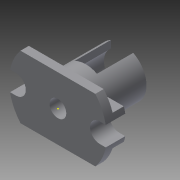
# Autodesk Inventor part: 零件6-23
Saved by Autodesk Inventor 2014 (Build 180170000, 170)
## iProperties
Created: 2018-11-23
Part Number: 零件6-23
Material: 常规
Document SubType Name: Modeling
Designer: Administrator
Density: 1 g/cm^3
Appearance: 默认
Author: Administrator
Autodesk Inventor part; units mm, degrees
ref_plane "YZ Plane" through (0, 0, 0) normal (1, 0, 0) x (0, 1, 0)
ref_plane "XZ Plane" through (0, 0, 0) normal (0, 1, 0) x (-1, 0, 0)
ref_plane "XY Plane" through (0, 0, 0) normal (0, 0, 1) x (1, 0, 0)
sketch "草图1" plane through (0, 0, 0) normal (0, 1, 0) x (-1, 0, 0)
  line L0 (55.7629, 0) -> (-64.7988, 0)
  line L1 (26.8095, -22.5) -> (-26.8095, -22.5)
  line L2 (26.8095, 22.5) -> (-29.1705, 22.5)
  line L3 (0, -45.1984) -> (0, 63.6584)
  arc A0 (30, 7) -> (30, -7) centre (30, 0) ccw
  arc A1 (-30, -7) -> (-30, 7) centre (-30, 0) ccw
  line L4 (30, -7) -> (34.2929, -7)
  line L5 (30, 7) -> (34.2929, 7)
  line L6 (-30, -7) -> (-34.2929, -7)
  line L7 (-30, 7) -> (-34.2929, 7)
  arc A2 (26.8095, -22.5) -> (34.2929, -7) centre (0, 0) ccw
  arc A3 (34.2929, 7) -> (26.8095, 22.5) centre (0, 0) ccw
  arc A4 (-26.8095, 22.5) -> (-34.2929, 7) centre (0, 0) ccw
  arc A5 (-34.2929, -7) -> (-26.8095, -22.5) centre (0, 0) ccw
  dimension "d1" = 45
  dimension "d2" = 14
  dimension "d3" = 60
  constraints: 16 end point, 12 point on circle, 6 centre point, 5 parallel, 5 point on line, 4 tangent, 2 perpendicular, 1 coincident, 1 horizontal, 2 other
  measures "d1" diameter of L1 L0
  measures "d2" diameter of A0
  measures "d3" distance of A1.centre A0.centre
extrude "拉伸1" add sketch "草图1" along normal blind 6
sketch "草图2" plane through (0, 6, 0) normal (0, 1, 0) x (1, 0, 0)
  arc A0 (34.2929, 7) -> (26.8095, 22.5) centre (0, 0) ccw projected
  circle A1 centre (0, 0) radius 17.5
  dimension "d6" = 35
  constraints: 1 centre point, 1 coincident
  measures "d6" diameter of A1
extrude "拉伸2" add sketch "草图2" along normal blind 40
sketch "草图3" plane through (0, 0, 0) normal (0, -1, 0) x (1, 0, 0)
  arc A0 (-34.2929, -7) -> (-26.8095, -22.5) centre (0, 0) ccw projected
  circle A1 centre (0, 0) radius 6
  dimension "d9" = 12
  constraints: 1 centre point, 1 coincident
  measures "d9" diameter of A1
extrude "拉伸3" cut sketch "草图3" against normal blind 60
sketch "草图4" plane through (0, 6, 0) normal (0, 1, 0) x (1, 0, 0)
  circle A0 centre (0, 0) radius 17.5 projected
  arc A1 (-26.8095, 22.5) -> (-34.2929, 7) centre (0, 0) ccw projected
  line L0 (-34.2929, 7) -> (-30, 7) projected
  arc A2 (-30, -7) -> (-30, 7) centre (-30, 0) ccw projected
  line L1 (-30, -7) -> (-34.2929, -7) projected
  arc A3 (-34.2929, -7) -> (-26.8095, -22.5) centre (0, 0) ccw projected
  arc A4 (26.8095, -22.5) -> (34.2929, -7) centre (0, 0) ccw projected
  line L2 (34.2929, -7) -> (30, -7) projected
  arc A5 (30, 7) -> (30, -7) centre (30, 0) ccw projected
  line L3 (30, 7) -> (34.2929, 7) projected
  arc A6 (34.2929, 7) -> (26.8095, 22.5) centre (0, 0) ccw projected
  line L4 (-33.2265, 11) -> (-13.6107, 11)
  line L5 (13.6107, 11) -> (33.2265, 11)
  line L6 (-33.2265, -11) -> (-13.6107, -11)
  line L7 (13.6107, -11) -> (33.2265, -11)
  line L8 (-37.479, 0) -> (55.827, 0)
  line L9 (0, 23.5503) -> (0, -22.0958)
  dimension "d12" = 22
  constraints: 12 end point, 8 point on circle, 3 parallel, 1 collinear, 1 perpendicular, 2 other
  measures "d12" diameter of L4 L8
extrude "拉伸4" add sketch "草图4" along normal blind 8 contours L8 A5 L2 A4 L7 A0 | A0 L5 A6 L3 A5 L8 | L8 A2 L0 A1 L4 A0 | A0 L6 A3 L1 A2 L8
sketch "草图5" plane through (0, 46, 0) normal (0, 1, 0) x (1, 0, 0)
  circle A0 centre (0, 0) radius 6 projected
  circle A1 centre (0, 0) radius 17.5 projected
  circle A2 centre (0, 0) radius 13
  dimension "d15" = 26
  constraints: 1 centre point, 1 coincident
  measures "d15" diameter of A2
extrude "拉伸5" cut sketch "草图5" against normal blind 26 contours A2
sketch "草图6" plane through (0, 0, 0) normal (0, 0, 1) x (1, 0, 0)
  point P0 (0, 0)
sketch "草图7" plane through (0, 0, 0) normal (0, 0, 1) x (1, 0, 0)
  line L0 (0, 0) -> (0, 58.8844)
  line L1 (-23, 14) -> (-17.5, 14) projected
  line L2 (-17.5, 14) -> (-17.5, 46) projected
  line L3 (-17.5, 46) -> (-13, 46) projected
  line L4 (-13, 46) -> (-13, 20) projected
  line L5 (-13, 20) -> (-6, 20) projected
  line L6 (-6, 20) -> (-6, 0) projected
  line L7 (-6, 0) -> (-23, 0) projected
  line L8 (-23, 0) -> (-23, 14) projected
  line L9 (17.5, 14) -> (23, 14) projected
  line L10 (23, 14) -> (23, 0) projected
  line L11 (23, 0) -> (6, 0) projected
  line L12 (6, 0) -> (6, 20) projected
  line L13 (6, 20) -> (13, 20) projected
  line L14 (13, 20) -> (13, 46) projected
  line L15 (13, 46) -> (17.5, 46) projected
  line L16 (17.5, 46) -> (17.5, 14) projected
  circle A0 centre (0, 34) radius 8
  line L17 (-13, 46) -> (13, 46) projected
  dimension "d18" = 16
  dimension "d19" = 12
  constraints: 2 end point, 1 centre point, 1 point on line, 1 vertical
  measures "d18" diameter of A0
  measures "d19" distance from line of L17 A0.centre
extrude "拉伸6" cut sketch "草图7" against normal blind 26 contours A0 L0 | L0 A0
sketch "草图8" plane through (0, 0, 0) normal (0, 0, 1) x (1, 0, 0)
  line L0 (-23, 14) -> (-17.5, 14) projected
  line L1 (-17.5, 14) -> (-17.5, 46) projected
  line L2 (-17.5, 46) -> (-13, 46) projected
  line L3 (-13, 46) -> (-13, 20) projected
  line L4 (-13, 20) -> (-6, 20) projected
  line L5 (-6, 20) -> (-6, 0) projected
  line L6 (-6, 0) -> (-23, 0) projected
  line L7 (-23, 0) -> (-23, 14) projected
  line L8 (17.5, 14) -> (23, 14) projected
  line L9 (23, 14) -> (23, 0) projected
  line L10 (23, 0) -> (6, 0) projected
  line L11 (6, 0) -> (6, 20) projected
  line L12 (6, 20) -> (13, 20) projected
  line L13 (13, 20) -> (13, 46) projected
  line L14 (13, 46) -> (17.5, 46) projected
  line L15 (17.5, 46) -> (17.5, 14) projected
  line L16 (-23, 14) -> (-17.5, 14) projected
  line L17 (-17.5, 14) -> (-17.5, 46) projected
  line L18 (-17.5, 46) -> (-13, 46) projected
  line L19 (-13, 46) -> (-13, 20) projected
  line L20 (-13, 20) -> (-6, 20) projected
  line L21 (-6, 20) -> (-6, 0) projected
  line L22 (-6, 0) -> (-23, 0) projected
  line L23 (-23, 0) -> (-23, 14) projected
  line L24 (17.5, 14) -> (23, 14) projected
  line L25 (23, 14) -> (23, 0) projected
  line L26 (23, 0) -> (6, 0) projected
  line L27 (6, 0) -> (6, 20) projected
  line L28 (6, 20) -> (13, 20) projected
  line L29 (13, 20) -> (13, 46) projected
  line L30 (13, 46) -> (17.5, 46) projected
  line L31 (17.5, 46) -> (17.5, 14) projected
  line L32 (-23, 14) -> (-17.5, 14) projected
  line L33 (-17.5, 14) -> (-17.5, 46) projected
  line L34 (-17.5, 46) -> (-13, 46) projected
  line L35 (-13, 46) -> (-13, 20) projected
  line L36 (-13, 20) -> (-6, 20) projected
  line L37 (-6, 20) -> (-6, 0) projected
  line L38 (-6, 0) -> (-23, 0) projected
  line L39 (-23, 0) -> (-23, 14) projected
  line L40 (17.5, 14) -> (23, 14) projected
  line L41 (23, 14) -> (23, 0) projected
  line L42 (23, 0) -> (6, 0) projected
  line L43 (6, 0) -> (6, 20) projected
  line L44 (6, 20) -> (13, 20) projected
  line L45 (13, 20) -> (13, 46) projected
  line L46 (13, 46) -> (17.5, 46) projected
  line L47 (17.5, 46) -> (17.5, 14) projected
  line L48 (0, 49.6225) -> (0, -12.8831)
  line L49 (-8, 46) -> (8, 46)
  line L50 (8, 46) -> (8, 20)
  line L51 (8, 20) -> (-8, 20)
  line L52 (-8, 20) -> (-8, 46)
  point P0 (0, 0)
  dimension "d22" = 16
  dimension "d23" = 26
  constraints: 10 end point, 3 parallel, 1 horizontal, 1 perpendicular, 1 point on line, 1 other
  measures "d22" distance of L50.end L51.end
  measures "d23" distance of L51.end L49.start
extrude "拉伸7" cut sketch "草图8" along normal blind 26 contours L4 L52 L49 L48 L51 | L48 L49 L50 L12 L51
